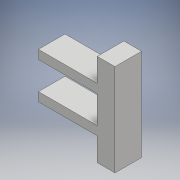
# Autodesk Inventor part: haut support
Saved by Autodesk Inventor 2018 (Build 220112000, 112)
## iProperties
Created: 2018-05-22
Part Number: haut support
Material: Générique
Document SubType Name: Modeling
Designer: Dimitri
Density: 1 g/cm^3
Appearance: Par défaut
Author: Dimitri
Autodesk Inventor part; units mm, degrees
ref_plane "YZ Plane" through (0, 0, 0) normal (1, 0, 0) x (0, 1, 0)
ref_plane "XZ Plane" through (0, 0, 0) normal (0, 1, 0) x (-1, 0, 0)
ref_plane "XY Plane" through (0, 0, 0) normal (0, 0, 1) x (1, 0, 0)
sketch "Esquisse1" plane through (0, 0, 0) normal (0, 1, 0) x (-1, 0, 0)
  line L0 (89.3861, -273.097) -> (89.3861, -280.097)
  line L1 (89.3861, -250.597) -> (89.3861, -263.7609)
  line L2 (89.3861, -302.597) -> (79.3861, -302.597)
  line L3 (79.3861, -302.597) -> (79.3861, -250.597)
  line L4 (122.5932, -263.7609) -> (89.3861, -263.7609)
  line L5 (89.3861, -268.7609) -> (122.5932, -268.7609)
  line L6 (122.5932, -289.4332) -> (89.3861, -289.4332)
  line L7 (89.3861, -284.4332) -> (122.5932, -284.4332)
  line L8 (89.3861, -289.4332) -> (89.3861, -302.597)
  line L9 (89.3861, -268.7609) -> (89.3861, -284.4332)
  line L10 (79.3861, -250.597) -> (89.3861, -250.597)
  line L11 (122.5932, -263.7609) -> (122.5932, -268.7609)
  line L12 (122.5932, -284.4332) -> (122.5932, -289.4332)
  point P0 (0, 0)
  dimension "d0" = 10
  dimension "d1" = 5
  dimension "d2" = 5
  constraints: 26 end point, 6 perpendicular, 1 point on line, 1 vertical
  measures "d0" distance of L8.end L3.start
  measures "d1" distance of L1.end L9.start
  measures "d2" distance of L6.end L9.end
extrude "Extrusion1" add sketch "Esquisse1" along normal blind 15
